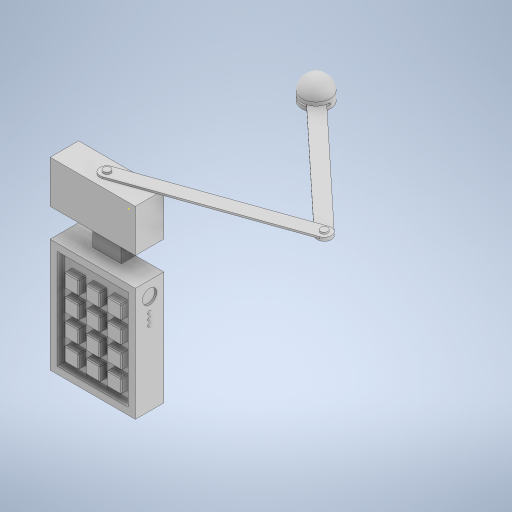
# Autodesk Inventor part: Weighted Door Closer
Saved by Autodesk Inventor 2024 (Build 280153000, 153)
## iProperties
Created: 2023-11-29
Part Number: Weighted Door Closer
Material: Generic
Document SubType Name: Modeling
Designer: ahale
Density: 1 g/cm^3
Appearance: Default
Author: ahale
Autodesk Inventor part; units mm, degrees
ref_plane "YZ Plane" through (0, 0, 0) normal (1, 0, 0) x (0, 1, 0)
ref_plane "XZ Plane" through (0, 0, 0) normal (0, 1, 0) x (-1, 0, 0)
ref_plane "XY Plane" through (0, 0, 0) normal (0, 0, 1) x (1, 0, 0)
sketch "Sketch2" plane through (0, 0, 0) normal (0, 1, 0) x (-1, 0, 0)
  circle A0 centre (0, 0) radius 25.4
  dimension "d4" = 50.8
  constraints: 1 centre point, 1 coincident
  measures "d4" diameter of A0
extrude "Extrusion2" add sketch "Sketch2" along normal blind 41.275
fillet "Fillet1" radius 25.4 1 edges at (25.4, 41.275, 0)
sketch "Sketch3" plane through (0, 0, 0) normal (1, 0, 0) x (0, 1, 0)
  line L0 (0, 25.4) -> (15.875, 25.4) projected
  line L1 (6.35, 0) -> (9.525, 0)
  line L2 (9.525, 0) -> (9.525, 25.4)
  line L3 (9.525, 25.4) -> (6.35, 25.4)
  line L4 (6.35, 25.4) -> (6.35, 0)
  line L5 (0, 35.56) -> (0, -35.56) projected
  point P0 (0, 0)
  dimension "d8" = 3.175
  dimension "d9" = 6.35
  constraints: 8 end point, 2 parallel, 1 horizontal, 1 perpendicular, 1 point on line
  measures "d8" distance between parallel lines of L4 L2
  measures "d9" distance between parallel lines of L5 L4
extrude "Extrusion3" cut sketch "Sketch3" along normal mid plane 127
sketch "Sketch5" plane through (0, 6.35, 0) normal (0, 1, 0) x (1, 0, 0)
  line L0 (0, 0) -> (222.7111, -208.0932) construction
  line L1 (-8.6706, -9.2796) -> (214.0406, -217.3729)
  line L2 (231.3817, -198.8136) -> (8.6706, 9.2796)
  arc A0 (8.6706, 9.2796) -> (-8.6706, -9.2796) centre (0, 0) ccw
  arc A1 (214.0406, -217.3729) -> (231.3817, -198.8136) centre (222.7111, -208.0932) ccw
  point P0 (111.3556, -104.0466)
  dimension "d16" = 304.8
  dimension "d17" = 25.4
  constraints: 8 end point, 4 point on circle, 4 tangent, 2 centre point, 1 midpoint, 1 parallel
  measures "d16" distance of L0.start L0.end
  measures "d17" diameter of A1
extrude "Extrusion5" add sketch "Sketch5" along normal blind 3.175
sketch "Sketch6" plane through (0, 9.525, 0) normal (0, 1, 0) x (1, 0, 0)
  arc A0 (214.0406, -217.3729) -> (231.3817, -198.8136) centre (222.7111, -208.0932) ccw projected
  line L0 (222.7111, -208.0932) -> (-64.656, -309.6963) construction
  line L1 (218.4777, -196.1196) -> (-68.8895, -297.7226)
  line L2 (-60.4225, -321.6699) -> (226.9446, -220.0669)
  arc A1 (226.9446, -220.0669) -> (218.4777, -196.1196) centre (222.7111, -208.0932) ccw
  arc A2 (-68.8895, -297.7226) -> (-60.4225, -321.6699) centre (-64.656, -309.6963) ccw
  point P0 (0, 0)
  point P1 (79.0276, -258.8948)
  dimension "d20" = 304.8
  dimension "d21" = 25.4
  constraints: 8 end point, 4 point on circle, 4 tangent, 2 centre point, 1 midpoint, 1 parallel
  measures "d20" distance of L0.start L0.end
  measures "d21" diameter of A2
extrude "Extrusion6" add sketch "Sketch6" along normal blind 3.175
sketch "Sketch7" plane through (0, 12.7, 0) normal (0, 1, 0) x (1, 0, 0)
  arc A0 (-68.8895, -297.7226) -> (-60.4225, -321.6699) centre (-64.656, -309.6963) ccw projected
  circle A1 centre (-64.656, -309.6963) radius 6.35
  point P0 (0, 0)
  dimension "d24" = 12.7
  constraints: 1 centre point, 1 coincident
  measures "d24" diameter of A1
extrude "Extrusion7" add sketch "Sketch7" along normal blind 3.175 and the other way blind 22.225
sketch "Sketch8" plane through (0, 12.7, 0) normal (0, 1, 0) x (1, 0, 0)
  arc A0 (226.9446, -220.0669) -> (218.4777, -196.1196) centre (222.7111, -208.0932) ccw projected
  circle A1 centre (222.7111, -208.0932) radius 6.35
  point P0 (0, 0)
  dimension "d29" = 12.7
  constraints: 1 centre point, 1 coincident
  measures "d29" diameter of A1
extrude "Extrusion8" add sketch "Sketch8" along normal blind 3.175 and the other way blind 9.525
sketch "Sketch9" plane through (0, 9.525, 0) normal (0, -1, 0) x (1, 0, 0)
  line L0 (-140.856, 284.2963) -> (11.544, 284.2963)
  line L1 (11.544, 284.2963) -> (11.544, 335.0963)
  line L2 (11.544, 335.0963) -> (-140.856, 335.0963)
  line L3 (-140.856, 335.0963) -> (-140.856, 284.2963)
  circle A0 centre (-64.656, 309.6963) radius 6.35 projected
  line L4 (-140.856, 284.2963) -> (11.544, 335.0963) construction
  line L5 (11.544, 284.2963) -> (-140.856, 335.0963) construction
  point P0 (0, 0)
  dimension "d34" = 152.4
  dimension "d35" = 50.8
  constraints: 12 end point, 2 midpoint, 2 parallel, 1 horizontal, 1 perpendicular
  measures "d34" distance of L2.end L1.end
  measures "d35" distance of L2.end L0.start
extrude "Extrusion9" add sketch "Sketch9" along normal blind 76.2 contours L3 L2 L1 L0 | A0
sketch "Sketch11" plane through (0, -66.675, 0) normal (0, -1, 0) x (1, 0, 0)
  line L0 (-90.056, 309.6963) -> (-90.056, 284.2963)
  line L1 (-90.056, 284.2963) -> (-39.256, 284.2963)
  line L2 (-39.256, 284.2963) -> (-39.256, 309.6963)
  line L3 (-39.256, 309.6963) -> (-90.056, 309.6963)
  line L4 (-90.056, 309.6963) -> (-90.056, 284.2963)
  line L5 (-140.856, 335.0963) -> (-140.856, 284.2963) projected
  line L6 (11.544, 335.0963) -> (-140.856, 335.0963) projected
  point P0 (0, 0)
  dimension "d41" = 50.8
  dimension "d42" = 25.4
  dimension "d45" = 50.8
  dimension "d46" = 25.4
  constraints: 10 end point, 2 parallel, 1 horizontal, 1 perpendicular
  measures "d41" distance of L3.end L2.end
  measures "d42" distance of L1.end L2.end
  measures "d45" distance between parallel lines of L5 L0
  measures "d46" distance between parallel lines of L6 L3
extrude "Extrusion10" add sketch "Sketch11" along normal blind 50.8
sketch "Sketch12" plane through (0, -117.475, 0) normal (0, -1, 0) x (1, 0, 0)
  line L0 (11.544, 335.0963) -> (-140.856, 335.0963) projected
  line L1 (11.544, 296.225) -> (11.544, 284.2963) projected
  line L2 (-140.856, 335.0963) -> (11.544, 335.0963)
  line L3 (11.544, 335.0963) -> (11.544, 284.2963)
  line L4 (11.544, 284.2963) -> (-140.856, 284.2963)
  line L5 (-140.856, 284.2963) -> (-140.856, 335.0963)
  point P0 (0, 0)
  constraints: 8 end point, 2 parallel, 1 horizontal, 1 perpendicular
extrude "Extrusion11" add sketch "Sketch12" along normal blind 203.2
sketch "Sketch13" plane through (-140.856, -117.475, 335.0963) normal (0, 0, 1) x (1, 0, 0)
  point P0 (140.856, 117.475)
sketch "Sketch14" plane through (-140.856, -117.475, 335.0963) normal (0, 0, 1) x (1, 0, 0)
  line L0 (12.7, -190.5) -> (139.7, -190.5)
  line L1 (139.7, -190.5) -> (139.7, -12.7)
  line L2 (139.7, -12.7) -> (12.7, -12.7)
  line L3 (12.7, -12.7) -> (12.7, -190.5)
  line L4 (12.7, -190.5) -> (139.7, -12.7) construction
  line L5 (139.7, -190.5) -> (12.7, -12.7) construction
  line L6 (152.4, 0) -> (0, 0) projected
  line L7 (0, 0) -> (0, -203.2) projected
  point P0 (140.856, 117.475)
  point P1 (76.2, -101.6)
  dimension "d51" = 127
  dimension "d52" = 177.8
  dimension "d53" = 101.6
  dimension "d54" = 76.2
  constraints: 12 end point, 2 midpoint, 2 parallel, 1 horizontal, 1 perpendicular
  measures "d51" distance of L2.end L1.end
  measures "d52" distance of L0.end L1.end
  measures "d53" distance from line of L6 point (76.2, -101.6)
  measures "d54" distance from line of L7 point (76.2, -101.6)
extrude "Extrusion12" cut sketch "Sketch14" against normal blind 12.7
sketch "Sketch15" plane through (-140.856, -117.475, 322.3963) normal (0, 0, 1) x (1, 0, 0)
  line L0 (25.4, -177.8) -> (50.8, -177.8)
  line L1 (50.8, -177.8) -> (50.8, -152.4)
  line L2 (50.8, -152.4) -> (25.4, -152.4)
  line L3 (25.4, -152.4) -> (25.4, -177.8)
  line L4 (12.7, -190.5) -> (12.7, -12.7) projected
  line L5 (139.7, -190.5) -> (12.7, -190.5) projected
  line L6 (88.9, -152.4) -> (63.5, -152.4)
  line L7 (63.5, -152.4) -> (63.5, -177.8)
  line L8 (63.5, -177.8) -> (88.9, -177.8)
  line L9 (88.9, -177.8) -> (88.9, -152.4)
  line L10 (127, -152.4) -> (101.6, -152.4)
  line L11 (101.6, -152.4) -> (101.6, -177.8)
  line L12 (101.6, -177.8) -> (127, -177.8)
  line L13 (127, -177.8) -> (127, -152.4)
  line L14 (50.8, -114.3) -> (25.4, -114.3)
  line L15 (25.4, -114.3) -> (25.4, -139.7)
  line L16 (25.4, -139.7) -> (50.8, -139.7)
  line L17 (50.8, -139.7) -> (50.8, -114.3)
  line L18 (88.9, -114.3) -> (63.5, -114.3)
  line L19 (63.5, -114.3) -> (63.5, -139.7)
  line L20 (63.5, -139.7) -> (88.9, -139.7)
  line L21 (88.9, -139.7) -> (88.9, -114.3)
  line L22 (127, -114.3) -> (101.6, -114.3)
  line L23 (101.6, -114.3) -> (101.6, -139.7)
  line L24 (101.6, -139.7) -> (127, -139.7)
  line L25 (127, -139.7) -> (127, -114.3)
  line L26 (50.8, -76.2) -> (25.4, -76.2)
  line L27 (25.4, -76.2) -> (25.4, -101.6)
  line L28 (25.4, -101.6) -> (50.8, -101.6)
  line L29 (50.8, -101.6) -> (50.8, -76.2)
  line L30 (88.9, -76.2) -> (63.5, -76.2)
  line L31 (63.5, -76.2) -> (63.5, -101.6)
  line L32 (63.5, -101.6) -> (88.9, -101.6)
  line L33 (88.9, -101.6) -> (88.9, -76.2)
  line L34 (127, -76.2) -> (101.6, -76.2)
  line L35 (101.6, -76.2) -> (101.6, -101.6)
  line L36 (101.6, -101.6) -> (127, -101.6)
  line L37 (127, -101.6) -> (127, -76.2)
  line L38 (50.8, -38.1) -> (25.4, -38.1)
  line L39 (25.4, -38.1) -> (25.4, -63.5)
  line L40 (25.4, -63.5) -> (50.8, -63.5)
  line L41 (50.8, -63.5) -> (50.8, -38.1)
  line L42 (88.9, -38.1) -> (63.5, -38.1)
  line L43 (63.5, -38.1) -> (63.5, -63.5)
  line L44 (63.5, -63.5) -> (88.9, -63.5)
  line L45 (88.9, -63.5) -> (88.9, -38.1)
  line L46 (127, -38.1) -> (101.6, -38.1)
  line L47 (101.6, -38.1) -> (101.6, -63.5)
  line L48 (101.6, -63.5) -> (127, -63.5)
  line L49 (127, -63.5) -> (127, -38.1)
  point P0 (140.856, 117.475)
  dimension "d57" = 12.7
  dimension "d58" = 12.7
  dimension "d59" = 25.4
  dimension "d60" = 25.4
  dimension "d63" = 38.1
  dimension "d66" = 38.1
  constraints: 96 end point, 2 horizontal, 2 parallel, 1 perpendicular, 1 vertical, 88 other
  measures "d57" distance between parallel lines of L4 L3
  measures "d58" distance between parallel lines of L5 L0
  measures "d59" distance between parallel lines of L1 L3
  measures "d60" distance of L0.end L1.end
  measures "d63" distance of L1.end L6.start
  measures "d66" distance of L1.end L14.start
extrude "Extrusion13" add sketch "Sketch15" along normal blind 12.7
sketch "Sketch16" plane through (11.544, -117.475, 335.0963) normal (1, 0, 0) x (0, 0, -1)
  circle A0 centre (25.4, -25.4) radius 12.7
  circle A1 centre (25.4, -50.8) radius 3.175
  line L0 (50.8, 0) -> (0, 0) projected
  line L1 (50.8, 0) -> (50.8, -203.2) projected
  circle A2 centre (25.4, -60.325) radius 3.175
  circle A3 centre (25.4, -69.85) radius 3.175
  point P0 (335.0963, 117.475)
  dimension "d71" = 25.4
  dimension "d72" = 6.35
  dimension "d73" = 25.4
  dimension "d75" = 25.4
  dimension "d79" = 9.525
  constraints: 4 centre point, 1 vertical, 4 other
  measures "d71" diameter of A0
  measures "d72" diameter of A1
  measures "d73" distance from line of L0 A0.centre
  measures "d75" distance from line of L1 A0.centre
  measures "d79" distance of A1.centre A2.centre
extrude "Extrusion14" cut sketch "Sketch16" against normal blind 3.175 contours A0
sketch "Sketch17" plane through (11.544, -117.475, 335.0963) normal (1, 0, 0) x (0, 0, -1)
  circle A0 centre (25.4, -50.8) radius 3.175
  line L0 (50.8, 0) -> (0, 0) projected
  line L1 (50.8, 0) -> (50.8, -203.2) projected
  circle A1 centre (25.4, -60.325) radius 3.175
  circle A2 centre (25.4, -69.85) radius 3.175
  point P0 (335.0963, 117.475)
  dimension "d86" = 6.35
  dimension "d87" = 50.8
  dimension "d88" = 25.4
  dimension "d91" = 9.525
  constraints: 3 centre point, 1 vertical, 4 other
  measures "d86" diameter of A0
  measures "d87" distance from line of L0 A0.centre
  measures "d88" distance from line of L1 A0.centre
  measures "d91" distance of A0.centre A1.centre
extrude "Extrusion15" add sketch "Sketch17" along normal blind 3.175
fillet "Fillet3" radius 3.175 3 edges at (14.719, -168.275, 312.8713) (14.719, -177.8, 312.8713) (14.719, -187.325, 312.8713)
fillet "Fillet4" radius 1.5875 51 edges at (-102.756, -155.575, 335.0963) (-115.456, -155.575, 328.7463) (-115.456, -168.275, 335.0963) (-102.756, -180.975, 335.0963) (-115.456, -180.975, 328.7463) (-115.456, -193.675, 328.7463) (-115.456, -219.075, 328.7463) (-115.456, -231.775, 328.7463) (-115.456, -257.175, 328.7463) (-115.456, -269.875, 328.7463) (-115.456, -295.275, 328.7463) (-102.756, -295.275, 335.0963) (-115.456, -282.575, 335.0963) (-102.756, -269.875, 335.0963) (-102.756, -257.175, 335.0963) (-102.756, -231.775, 335.0963) (-102.756, -219.075, 335.0963) (-102.756, -193.675, 335.0963) (-115.456, -206.375, 335.0963) (-115.456, -244.475, 335.0963) (-90.056, -168.275, 335.0963) (-90.056, -155.575, 328.7463) (-90.056, -180.975, 328.7463) (-77.356, -168.275, 335.0963) (-51.956, -168.275, 335.0963) (-39.256, -168.275, 335.0963) (-13.856, -168.275, 335.0963) (-13.856, -206.375, 335.0963) (-39.256, -206.375, 335.0963) (-51.956, -206.375, 335.0963) (-77.356, -206.375, 335.0963) (-90.056, -244.475, 335.0963) (-77.356, -244.475, 335.0963) (-51.956, -244.475, 335.0963) (-39.256, -244.475, 335.0963) (-13.856, -244.475, 335.0963) (-77.356, -282.575, 335.0963) (-90.056, -282.575, 335.0963) (-51.956, -282.575, 335.0963) (-39.256, -282.575, 335.0963) (-13.856, -282.575, 335.0963) (-26.556, -295.275, 335.0963) (-26.556, -269.875, 335.0963) (-26.556, -257.175, 335.0963) (-26.556, -231.775, 335.0963) (-26.556, -219.075, 335.0963) (-26.556, -193.675, 335.0963) (-26.556, -180.975, 335.0963) (-26.556, -155.575, 335.0963) (-64.656, -155.575, 335.0963) (-64.656, -180.975, 335.0963)
fillet "Fillet5" radius 1.5875 44 edges at (-90.056, -194.14, 334.6313) (-90.056, -193.675, 327.9525) (-90.056, -218.61, 334.6313) (-90.056, -219.075, 327.9525) (-90.056, -206.375, 335.0963) (-76.891, -193.675, 334.6313) (-77.356, -193.675, 327.9525) (-52.421, -193.675, 334.6313) (-51.956, -193.675, 327.9525) (-64.656, -193.675, 335.0963) (-52.421, -156.04, 334.6313) (-51.956, -155.575, 327.9525) (-76.891, -156.04, 334.6313) (-77.356, -155.575, 327.9525) (-52.421, -180.51, 334.6313) (-51.956, -180.975, 327.9525) (-76.891, -180.51, 334.6313) (-77.356, -180.975, 327.9525) (-38.791, -180.51, 334.6313) (-39.256, -180.975, 327.9525) (-14.321, -180.51, 334.6313) (-13.856, -180.975, 327.9525) (-14.321, -156.04, 334.6313) (-13.856, -155.575, 327.9525) (-38.791, -156.04, 334.6313) (-39.256, -155.575, 327.9525) (-52.421, -219.075, 334.6313) (-51.956, -219.075, 327.9525) (-76.891, -219.075, 334.6313) (-77.356, -219.075, 327.9525) (-64.656, -219.075, 335.0963) (-52.421, -231.775, 334.6313) (-64.656, -231.775, 335.0963) (-76.891, -231.775, 334.6313) (-77.356, -231.775, 327.9525) (-51.956, -231.775, 327.9525) (-38.791, -194.14, 334.6313) (-39.256, -193.675, 327.9525) (-14.321, -194.14, 334.6313) (-13.856, -193.675, 327.9525) (-14.321, -218.61, 334.6313) (-13.856, -219.075, 327.9525) (-38.791, -218.61, 334.6313) (-39.256, -219.075, 327.9525)
fillet "Fillet6" radius 1.5875 24 edges at (-90.521, -256.71, 334.6313) (-90.056, -257.175, 327.9525) (-90.521, -270.34, 334.6313) (-90.056, -269.875, 327.9525) (-90.521, -294.81, 334.6313) (-90.056, -295.275, 327.9525) (-76.891, -295.275, 334.6313) (-64.656, -295.275, 335.0963) (-52.421, -295.275, 334.6313) (-51.956, -295.275, 327.9525) (-77.356, -295.275, 327.9525) (-76.891, -269.875, 334.6313) (-77.356, -269.875, 327.9525) (-52.421, -269.875, 334.6313) (-51.956, -269.875, 327.9525) (-64.656, -269.875, 335.0963) (-14.321, -294.81, 334.6313) (-13.856, -295.275, 327.9525) (-14.321, -270.34, 334.6313) (-13.856, -269.875, 327.9525) (-38.791, -270.34, 334.6313) (-39.256, -269.875, 327.9525) (-38.791, -294.81, 334.6313) (-39.256, -295.275, 327.9525)
body "Solid2"
